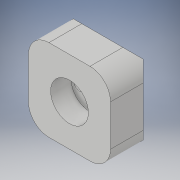
# Autodesk Inventor part: testled
Saved by Autodesk Inventor 2017 SP1 (Build 210196100, 196)
## iProperties
Created: 2016-12-24
Part Number: testled
Material: Generic
Document SubType Name: Modeling
Designer: wsh32
Density: 1 g/cm^3
Appearance: Default
Author: wsh32
Autodesk Inventor part; units mm, degrees
ref_plane "YZ Plane" through (0, 0, 0) normal (1, 0, 0) x (0, 1, 0)
ref_plane "XZ Plane" through (0, 0, 0) normal (0, 1, 0) x (-1, 0, 0)
ref_plane "XY Plane" through (0, 0, 0) normal (0, 0, 1) x (1, 0, 0)
sketch "Sketch1" plane through (0, 0, 0) normal (0, 0, 1) x (1, 0, 0)
  line L0 (0, 0) -> (12.7, 0)
  line L1 (12.7, 0) -> (12.7, 12.7)
  line L2 (12.7, 12.7) -> (0, 12.7)
  line L3 (0, 12.7) -> (0, 0)
  dimension "d0" = 12.7
  dimension "d1" = 12.7
  constraints: 8 end point, 2 parallel, 1 horizontal, 1 perpendicular
  measures "d0" distance of L2.end L0.start
  measures "d1" distance of L0.start L0.end
extrude "Extrusion1" add sketch "Sketch1" along normal blind 6.35
sketch "Sketch2" plane through (0, 0, 6.35) normal (0, 0, 1) x (1, 0, 0)
  line L0 (12.7, 12.7) -> (0, 12.7) construction
  line L1 (0, 0) -> (12.7, 0) construction
  line L2 (0, 12.7) -> (12.7, 0) construction
  line L3 (0, 0) -> (12.7, 12.7) construction
  circle A0 centre (6.35, 6.35) radius 2.921
  dimension "d4" = 5.842
  constraints: 4 end point, 1 centre point, 1 midpoint
  measures "d4" diameter of A0
extrude "Extrusion2" cut sketch "Sketch2" against normal blind 3.175
sketch "Sketch3" plane through (6.35, 6.35, 3.175) normal (0, 0, 1) x (1, 0, 0)
  circle A0 centre (0, 0) radius 2.921 construction
  line L0 (-6.35, 0) -> (6.35, 0) construction
  line L1 (-6.35, 6.35) -> (-6.35, -6.35) construction
  line L2 (6.35, -6.35) -> (6.35, 6.35) construction
  circle A1 centre (-1.5875, 0) radius 0.635 construction
  circle A2 centre (1.5875, 0) radius 0.635 construction
  line L3 (-0.9525, 6.35) -> (-0.9525, -6.35) construction
  line L4 (0.9525, -6.35) -> (0.9525, 6.35) construction
  point P0 (1.5875, 0)
  dimension "d7" = 1.27
  dimension "d8" = 1.27
  dimension "d9" = 1.5875
  dimension "d10" = 1.5875
  dimension "d11" = 1.905
  dimension "d26" = 3.175
  constraints: 6 end point, 2 centre point, 2 coincident, 2 equal length, 2 midpoint, 2 point on line, 2 symmetric about line, 2 tangent, 2 vertical
  measures "d7" diameter of A1
  measures "d8" diameter of A2
  measures "d9" distance of A0.centre point (-1.587, 0)
  measures "d10" distance of A0.centre A2.centre
  measures "d11" distance between parallel lines of L3 L4
  measures "d26" distance of A2.centre A1.centre
hole "Hole1" at (4.7625, 6.35, 3.175) at (7.9375, 6.35, 3.175) direction (0, 0, -1) diameter 1.905 end through all
chamfer "Chamfer2" distance 1.27 angle 45 4 edges at (6.35, 0, 0) (12.7, 6.35, 0) (6.35, 12.7, 0) (0, 6.35, 0)
fillet "Fillet1" radius 3.175 4 edges at (12.7, 0, 3.81) (12.7, 12.7, 3.81) (0, 12.7, 3.81) (0, 0, 3.81)
equation "\"d10\" = d9"
body "Solid1"
